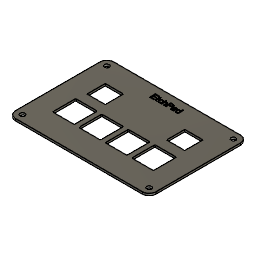
EtchPad_Case (Autodesk Fusion 360 archive; units mm, degrees)
design "EtchPad_Case_Top"
Autodesk Fusion 360 part; units mm, degrees
sketch "Sketch1" plane through (0, 0, 0) normal (0, 0, 1) x (1, 0, 0)
  line L0 (3.025, -31.1) -> (16.025, -31.1)
  line L1 (3.025, -45.1) -> (16.025, -45.1)
  line L2 (2.525, -31.6) -> (2.525, -44.6)
  line L3 (16.525, -31.6) -> (16.525, -44.6)
  arc A0 (3.025, -31.1) -> (2.525, -31.6) centre (3.025, -31.6) ccw
  arc A1 (16.525, -31.6) -> (16.025, -31.1) centre (16.025, -31.6) ccw
  arc A2 (2.525, -44.6) -> (3.025, -45.1) centre (3.025, -44.6) ccw
  arc A3 (16.025, -45.1) -> (16.525, -44.6) centre (16.025, -44.6) ccw
  line L4 (22.075, -31.1) -> (35.075, -31.1)
  line L5 (22.075, -45.1) -> (35.075, -45.1)
  line L6 (21.575, -31.6) -> (21.575, -44.6)
  line L7 (35.575, -31.6) -> (35.575, -44.6)
  arc A4 (22.075, -31.1) -> (21.575, -31.6) centre (22.075, -31.6) ccw
  arc A5 (35.575, -31.6) -> (35.075, -31.1) centre (35.075, -31.6) ccw
  arc A6 (21.575, -44.6) -> (22.075, -45.1) centre (22.075, -44.6) ccw
  arc A7 (35.075, -45.1) -> (35.575, -44.6) centre (35.075, -44.6) ccw
  line L8 (41.125, -31.1) -> (54.125, -31.1)
  line L9 (41.125, -45.1) -> (54.125, -45.1)
  line L10 (40.625, -31.6) -> (40.625, -44.6)
  line L11 (54.625, -31.6) -> (54.625, -44.6)
  arc A8 (41.125, -31.1) -> (40.625, -31.6) centre (41.125, -31.6) ccw
  arc A9 (54.625, -31.6) -> (54.125, -31.1) centre (54.125, -31.6) ccw
  arc A10 (40.625, -44.6) -> (41.125, -45.1) centre (41.125, -44.6) ccw
  arc A11 (54.125, -45.1) -> (54.625, -44.6) centre (54.125, -44.6) ccw
  line L12 (60.175, -31.1) -> (73.175, -31.1)
  line L13 (60.175, -45.1) -> (73.175, -45.1)
  line L14 (59.675, -31.6) -> (59.675, -44.6)
  line L15 (73.675, -31.6) -> (73.675, -44.6)
  arc A12 (60.175, -31.1) -> (59.675, -31.6) centre (60.175, -31.6) ccw
  arc A13 (73.675, -31.6) -> (73.175, -31.1) centre (73.175, -31.6) ccw
  arc A14 (59.675, -44.6) -> (60.175, -45.1) centre (60.175, -44.6) ccw
  arc A15 (73.175, -45.1) -> (73.675, -44.6) centre (73.175, -44.6) ccw
  line L16 (88.6, -63.6) -> (-12.4, -63.6)
  line L17 (-12.4, -63.6) -> (-12.4, 7)
  line L18 (-12.4, 7) -> (88.6, 7)
  line L19 (88.6, 7) -> (88.6, -63.6)
  line L20 (88.6, -63.6) -> (-12.4, 7) construction
  line L21 (-12.4, -63.6) -> (88.6, 7) construction
  line L22 (78.6, -53.6) -> (-2.4, -53.6)
  line L23 (-2.4, -53.6) -> (-2.4, -3)
  line L24 (-2.4, -3) -> (78.6, -3)
  line L25 (78.6, -3) -> (78.6, -53.6)
  circle A16 centre (-7.4, -58.6) radius 1.7
  circle A17 centre (83.6, 2) radius 1.7
  circle A18 centre (83.6, -58.6) radius 1.7
  circle A19 centre (-7.4, 2) radius 1.7
  point P0 (38.1, -28.3)
  dimension "d1" = 101
  dimension "d2" = 70.6
  dimension "d3" = 10
  dimension "d9" = 3.4
  dimension "d12" = 3.4
  dimension "d13" = 3.4
  dimension "d14" = 3.4
  constraint horizontal L16
  constraint perpendicular L16 L17
  constraint parallel L16 L18
  constraint parallel L17 L19
  constraint coincident L20 P0
  constraint coincident L21 P0
  measures "d1" distance of L17.end L18.end
  measures "d2" distance of L16.end L17.end
  measures "d9" diameter of A16
  measures "d12" diameter of A17
  measures "d13" diameter of A18
  measures "d14" diameter of A19
extrude "Extrude1" add sketch "Sketch1" along normal blind 1.5 contours L16 L17 L18 L19 | L22 L23 L24 L25
sketch "Sketch2" plane through (0, 0, 1.5) normal (0, 0, 1) x (-1, 0, 0)
  arc A0 (-41.125, 31.1) -> (-40.625, 31.6) centre (-41.125, 31.6) ccw
  line L0 (-41.125, 31.1) -> (-54.125, 31.1)
  arc A1 (-54.625, 31.6) -> (-54.125, 31.1) centre (-54.125, 31.6) ccw
  line L1 (-54.625, 31.6) -> (-54.625, 44.6)
  arc A2 (-54.125, 45.1) -> (-54.625, 44.6) centre (-54.125, 44.6) ccw
  line L2 (-54.125, 45.1) -> (-41.125, 45.1)
  arc A3 (-40.625, 44.6) -> (-41.125, 45.1) centre (-41.125, 44.6) ccw
  line L3 (-40.625, 44.6) -> (-40.625, 31.6)
  circle A4 centre (-83.6, 58.6) radius 1.7
  circle A5 centre (7.4, 58.6) radius 1.7
  arc A6 (-22.075, 31.1) -> (-21.575, 31.6) centre (-22.075, 31.6) ccw
  line L4 (-22.075, 31.1) -> (-35.075, 31.1)
  arc A7 (-35.575, 31.6) -> (-35.075, 31.1) centre (-35.075, 31.6) ccw
  line L5 (-35.575, 31.6) -> (-35.575, 44.6)
  arc A8 (-35.075, 45.1) -> (-35.575, 44.6) centre (-35.075, 44.6) ccw
  line L6 (-35.075, 45.1) -> (-22.075, 45.1)
  arc A9 (-21.575, 44.6) -> (-22.075, 45.1) centre (-22.075, 44.6) ccw
  line L7 (-21.575, 44.6) -> (-21.575, 31.6)
  arc A10 (-3.025, 31.1) -> (-2.525, 31.6) centre (-3.025, 31.6) ccw
  line L8 (-3.025, 31.1) -> (-16.025, 31.1)
  arc A11 (-16.525, 31.6) -> (-16.025, 31.1) centre (-16.025, 31.6) ccw
  line L9 (-16.525, 31.6) -> (-16.525, 44.6)
  arc A12 (-16.025, 45.1) -> (-16.525, 44.6) centre (-16.025, 44.6) ccw
  line L10 (-16.025, 45.1) -> (-3.025, 45.1)
  arc A13 (-2.525, 44.6) -> (-3.025, 45.1) centre (-3.025, 44.6) ccw
  line L11 (-2.525, 44.6) -> (-2.525, 31.6)
  arc A14 (-60.175, 31.1) -> (-59.675, 31.6) centre (-60.175, 31.6) ccw
  line L12 (-60.175, 31.1) -> (-73.175, 31.1)
  arc A15 (-73.675, 31.6) -> (-73.175, 31.1) centre (-73.175, 31.6) ccw
  line L13 (-73.675, 31.6) -> (-73.675, 44.6)
  arc A16 (-73.175, 45.1) -> (-73.675, 44.6) centre (-73.175, 44.6) ccw
  line L14 (-73.175, 45.1) -> (-60.175, 45.1)
  arc A17 (-59.675, 44.6) -> (-60.175, 45.1) centre (-60.175, 44.6) ccw
  line L15 (-59.675, 44.6) -> (-59.675, 31.6)
  circle A18 centre (-83.6, -2) radius 1.7
  circle A19 centre (7.4, -2) radius 1.7
  line L16 (-88.6, -7) -> (12.4, -7)
  line L17 (12.4, -7) -> (12.4, 63.6)
  line L18 (12.4, 63.6) -> (-88.6, 63.6)
  line L19 (-88.6, 63.6) -> (-88.6, -7)
  line L20 (-27.4431, 12.4012) -> (-48.7413, 12.4127) construction
  line L21 (-48.7413, 12.4127) -> (-48.7491, -1.9941) construction
  line L22 (-48.7491, -1.9941) -> (-27.4509, -2.0057) construction
  line L23 (-27.4509, -2.0057) -> (-27.4431, 12.4012) construction
  line L24 (-38.1, -2) -> (-38.1, -1.9999)
  dimension "d17" = 4
  dimension "d20" = 0.0001
  text T0 "EtchPad" font "Arial" height 4 align left top in box 21.2982 x 14.4068 at (-27.4431, 12.4012) x (-1, 0.000542) y (-0.000542, -1) spacing 1 kerned
  constraint midpoint L22 L24.end
  constraint vertical L24
  measures "d20" distance of L24.start L24.end
extrude "Extrude2" cut sketch "Sketch2" against normal blind 0.2 text T0
fillet "Fillet1" radius 5 4 edges at (-12.4, -63.6, 0.75) (88.6, -63.6, 0.75) (88.6, 7, 0.75) (-12.4, 7, 0.75)
sketch "Sketch3" plane through (0, 0, 1.5) normal (0, 0, 1) x (-1, 0, 0)
  arc A0 (7.4, -7) -> (12.4, -2) centre (7.4, -2) ccw
  line L0 (12.4, -2) -> (12.4, 58.6)
  arc A1 (12.4, 58.6) -> (7.4, 63.6) centre (7.4, 58.6) ccw
  line L1 (7.4, 63.6) -> (-83.6, 63.6)
  arc A2 (-83.6, 63.6) -> (-88.6, 58.6) centre (-83.6, 58.6) ccw
  line L2 (-88.6, 58.6) -> (-88.6, -2)
  arc A3 (-88.6, -2) -> (-83.6, -7) centre (-83.6, -2) ccw
  line L3 (-83.6, -7) -> (7.4, -7)
  circle A4 centre (7.4, -2) radius 1.7
  circle A5 centre (-83.6, -2) radius 1.7
  arc A6 (-60.175, 31.1) -> (-59.675, 31.6) centre (-60.175, 31.6) ccw
  line L4 (-60.175, 31.1) -> (-73.175, 31.1)
  arc A7 (-73.675, 31.6) -> (-73.175, 31.1) centre (-73.175, 31.6) ccw
  line L5 (-73.675, 31.6) -> (-73.675, 44.6)
  arc A8 (-73.175, 45.1) -> (-73.675, 44.6) centre (-73.175, 44.6) ccw
  line L6 (-73.175, 45.1) -> (-60.175, 45.1)
  arc A9 (-59.675, 44.6) -> (-60.175, 45.1) centre (-60.175, 44.6) ccw
  line L7 (-59.675, 44.6) -> (-59.675, 31.6)
  arc A10 (-3.025, 31.1) -> (-2.525, 31.6) centre (-3.025, 31.6) ccw
  line L8 (-3.025, 31.1) -> (-16.025, 31.1)
  arc A11 (-16.525, 31.6) -> (-16.025, 31.1) centre (-16.025, 31.6) ccw
  line L9 (-16.525, 31.6) -> (-16.525, 44.6)
  arc A12 (-16.025, 45.1) -> (-16.525, 44.6) centre (-16.025, 44.6) ccw
  line L10 (-16.025, 45.1) -> (-3.025, 45.1)
  arc A13 (-2.525, 44.6) -> (-3.025, 45.1) centre (-3.025, 44.6) ccw
  line L11 (-2.525, 44.6) -> (-2.525, 31.6)
  arc A14 (-22.075, 31.1) -> (-21.575, 31.6) centre (-22.075, 31.6) ccw
  line L12 (-22.075, 31.1) -> (-35.075, 31.1)
  arc A15 (-35.575, 31.6) -> (-35.075, 31.1) centre (-35.075, 31.6) ccw
  line L13 (-35.575, 31.6) -> (-35.575, 44.6)
  arc A16 (-35.075, 45.1) -> (-35.575, 44.6) centre (-35.075, 44.6) ccw
  line L14 (-35.075, 45.1) -> (-22.075, 45.1)
  arc A17 (-21.575, 44.6) -> (-22.075, 45.1) centre (-22.075, 44.6) ccw
  line L15 (-21.575, 44.6) -> (-21.575, 31.6)
  circle A18 centre (7.4, 58.6) radius 1.7
  circle A19 centre (-83.6, 58.6) radius 1.7
  arc A20 (-41.125, 31.1) -> (-40.625, 31.6) centre (-41.125, 31.6) ccw
  line L16 (-41.125, 31.1) -> (-54.125, 31.1)
  arc A21 (-54.625, 31.6) -> (-54.125, 31.1) centre (-54.125, 31.6) ccw
  line L17 (-54.625, 31.6) -> (-54.625, 44.6)
  arc A22 (-54.125, 45.1) -> (-54.625, 44.6) centre (-54.125, 44.6) ccw
  line L18 (-54.125, 45.1) -> (-41.125, 45.1)
  arc A23 (-40.625, 44.6) -> (-41.125, 45.1) centre (-41.125, 44.6) ccw
  line L19 (-40.625, 44.6) -> (-40.625, 31.6)
  line L20 (-30.434, 1.5239) -> (-30.4337, 1.9959)
  line L21 (-30.4337, 1.9959) -> (-27.4487, 1.9943)
  line L22 (-27.4487, 1.9943) -> (-27.4509, -2.0057)
  line L23 (-27.4509, -2.0057) -> (-30.3431, -2.0041)
  line L24 (-30.3431, -2.0041) -> (-30.3429, -1.5321)
  line L25 (-30.3429, -1.5321) -> (-27.98, -1.5334)
  line L26 (-27.98, -1.5334) -> (-27.9793, -0.3083)
  line L27 (-27.9793, -0.3083) -> (-30.1921, -0.3071)
  line L28 (-30.1921, -0.3071) -> (-30.1919, 0.1623)
  line L29 (-30.1919, 0.1623) -> (-27.979, 0.1611)
  line L30 (-27.979, 0.1611) -> (-27.9783, 1.5226)
  line L31 (-27.9783, 1.5226) -> (-30.434, 1.5239)
  spline S0 degree 3 poles (-33.8172, 1.6594) (-33.9088, 1.6529) (-34.087, 1.6402) (-34.2305, 1.534) (-34.3003, 1.4824) knots 0 0 0 0 0.026903 0.052406 0.052406 0.052406 0.052406
  spline S1 degree 3 poles (-34.3003, 1.4824) (-34.3596, 1.4104) (-34.4904, 1.2516) (-34.5265, 1.0481) (-34.5462, 0.9368) knots 0 0 0 0 0.027516 0.060744 0.060744 0.060744 0.060744
  line L32 (-34.5462, 0.9368) -> (-35.0291, 0.9998)
  spline S2 degree 3 poles (-35.0291, 0.9998) (-34.9949, 1.1549) (-34.9293, 1.4522) (-34.7224, 1.6748) (-34.6235, 1.7813) knots 0 0 0 0 0.046685 0.089485 0.089485 0.089485 0.089485
  spline S3 degree 3 poles (-34.6235, 1.7813) (-34.5065, 1.8636) (-34.2664, 2.0326) (-33.973, 2.0529) (-33.8225, 2.0633) knots 0 0 0 0 0.042047 0.086372 0.086372 0.086372 0.086372
  spline S4 degree 3 poles (-33.8225, 2.0633) (-33.636, 2.0492) (-33.2748, 2.0218) (-32.9995, 1.7874) (-32.8664, 1.6739) knots 0 0 0 0 0.054523 0.105641 0.105641 0.105641 0.105641
  spline S5 degree 3 poles (-32.8664, 1.6739) (-32.7612, 1.5213) (-32.5311, 1.1873) (-32.5145, 0.7802) (-32.5054, 0.5591) knots 0 0 0 0 0.054525 0.119313 0.119313 0.119313 0.119313
  spline S6 degree 3 poles (-32.5054, 0.5591) (-32.5106, 0.4109) (-32.5203, 0.129) (-32.616, -0.1362) (-32.6614, -0.2621) knots 0 0 0 0 0.044169 0.084044 0.084044 0.084044 0.084044
  spline S7 degree 3 poles (-32.6614, -0.2621) (-32.7192, -0.3715) (-32.8331, -0.5872) (-33.0355, -0.7229) (-33.1351, -0.7898) knots 0 0 0 0 0.036512 0.071907 0.071907 0.071907 0.071907
  spline S8 degree 3 poles (-33.1351, -0.7898) (-33.2439, -0.841) (-33.463, -0.9443) (-33.705, -0.9583) (-33.8269, -0.9654) knots 0 0 0 0 0.035714 0.071964 0.071964 0.071964 0.071964
  spline S9 degree 3 poles (-33.8269, -0.9654) (-33.9738, -0.9578) (-34.2521, -0.9434) (-34.4877, -0.7959) (-34.5989, -0.7262) knots 0 0 0 0 0.043319 0.082021 0.082021 0.082021 0.082021
  spline S10 degree 3 poles (-34.5989, -0.7262) (-34.6904, -0.6354) (-34.8816, -0.4456) (-34.9484, -0.1842) (-34.9833, -0.048) knots 0 0 0 0 0.037959 0.079265 0.079265 0.079265 0.079265
  line L33 (-34.9833, -0.048) -> (-34.5057, 0.0254)
  spline S11 degree 3 poles (-34.5057, 0.0254) (-34.4811, -0.0637) (-34.4352, -0.2297) (-34.3185, -0.3557) (-34.2645, -0.414) knots 0 0 0 0 0.027269 0.05078 0.05078 0.05078 0.05078
  spline S12 degree 3 poles (-34.2645, -0.414) (-34.2029, -0.457) (-34.0771, -0.5448) (-33.9239, -0.5559) (-33.8457, -0.5616) knots 0 0 0 0 0.022095 0.045141 0.045141 0.045141 0.045141
  spline S13 degree 3 poles (-33.8457, -0.5616) (-33.7284, -0.5512) (-33.4971, -0.5307) (-33.3266, -0.3734) (-33.2426, -0.2958) knots 0 0 0 0 0.03428 0.067589 0.067589 0.067589 0.067589
  spline S14 degree 3 poles (-33.2426, -0.2958) (-33.1752, -0.1842) (-33.0199, 0.0729) (-33.0137, 0.3749) (-33.0102, 0.5458) knots 0 0 0 0 0.038499 0.088664 0.088664 0.088664 0.088664
  spline S15 degree 3 poles (-33.0102, 0.5458) (-33.013, 0.7184) (-33.0179, 1.0214) (-33.1686, 1.2822) (-33.2335, 1.3945) knots 0 0 0 0 0.050719 0.089036 0.089036 0.089036 0.089036
  spline S16 degree 3 poles (-33.2335, 1.3945) (-33.3144, 1.4717) (-33.4779, 1.6279) (-33.7033, 1.6489) (-33.8172, 1.6594) knots 0 0 0 0 0.03254 0.06581 0.06581 0.06581 0.06581
  line L34 (-35.9407, 0.4137) -> (-35.9398, 1.9989)
  line L35 (-35.9398, 1.9989) -> (-35.4487, 1.9987)
  line L36 (-35.4487, 1.9987) -> (-35.4509, -2.0013)
  line L37 (-35.4509, -2.0013) -> (-35.942, -2.0011)
  line L38 (-35.942, -2.0011) -> (-35.9412, -0.5659)
  spline S17 degree 3 poles (-35.9412, -0.5659) (-36.0633, -0.682) (-36.3071, -0.9139) (-36.6419, -0.9472) (-36.8091, -0.9638) knots 0 0 0 0 0.049035 0.097945 0.097945 0.097945 0.097945
  spline S18 degree 3 poles (-36.8091, -0.9638) (-36.9109, -0.9595) (-37.1053, -0.9513) (-37.2835, -0.8736) (-37.3684, -0.8366) knots 0 0 0 0 0.030249 0.057797 0.057797 0.057797 0.057797
  spline S19 degree 3 poles (-37.3684, -0.8366) (-37.4414, -0.7912) (-37.584, -0.7025) (-37.6673, -0.5568) (-37.7079, -0.4858) knots 0 0 0 0 0.025355 0.049506 0.049506 0.049506 0.049506
  spline S20 degree 3 poles (-37.7079, -0.4858) (-37.7376, -0.3951) (-37.8064, -0.1846) (-37.8086, 0.0374) (-37.8099, 0.1637) knots 0 0 0 0 0.028475 0.066079 0.066079 0.066079 0.066079
  line L39 (-37.8099, 0.1637) -> (-37.8089, 1.9999)
  line L40 (-37.8089, 1.9999) -> (-37.3177, 1.9997)
  line L41 (-37.3177, 1.9997) -> (-37.3187, 0.1634)
  spline S21 degree 3 poles (-37.3187, 0.1634) (-37.3163, 0.0538) (-37.3118, -0.1407) (-37.2057, -0.3023) (-37.1594, -0.3729) knots 0 0 0 0 0.032071 0.056936 0.056936 0.056936 0.056936
  spline S22 degree 3 poles (-37.1594, -0.3729) (-37.0979, -0.4218) (-36.9663, -0.5264) (-36.7977, -0.5359) (-36.7079, -0.5409) knots 0 0 0 0 0.023016 0.04924 0.04924 0.04924 0.04924
  spline S23 degree 3 poles (-36.7079, -0.5409) (-36.6361, -0.5361) (-36.4915, -0.5265) (-36.3622, -0.4609) (-36.2972, -0.4279) knots 0 0 0 0 0.021368 0.04299 0.04299 0.04299 0.04299
  spline S24 degree 3 poles (-36.2972, -0.4279) (-36.2379, -0.3874) (-36.1212, -0.3076) (-36.0553, -0.1826) (-36.0229, -0.1211) knots 0 0 0 0 0.021195 0.041719 0.041719 0.041719 0.041719
  spline S25 degree 3 poles (-36.0229, -0.1211) (-35.999, -0.0448) (-35.9448, 0.129) (-35.9422, 0.3114) (-35.9407, 0.4137) knots 0 0 0 0 0.023859 0.054351 0.054351 0.054351 0.054351
  line L42 (-44.7857, 2.0037) -> (-44.2727, 2.0034)
  spline S26 degree 3 poles (-44.2727, 2.0034) (-44.2494, 1.9489) (-44.2005, 1.8342) (-44.1836, 1.7107) (-44.1747, 1.646) knots 0 0 0 0 0.017724 0.037217 0.037217 0.037217 0.037217
  spline S27 degree 3 poles (-44.1747, 1.646) (-44.0881, 1.7162) (-43.9264, 1.8471) (-43.7371, 1.9332) (-43.6493, 1.9731) knots 0 0 0 0 0.033289 0.062117 0.062117 0.062117 0.062117
  spline S28 degree 3 poles (-43.6493, 1.9731) (-43.5628, 2.0009) (-43.3866, 2.0575) (-43.2017, 2.0647) (-43.1076, 2.0683) knots 0 0 0 0 0.027122 0.055225 0.055225 0.055225 0.055225
  spline S29 degree 3 poles (-43.1076, 2.0683) (-42.9623, 2.0624) (-42.6951, 2.0516) (-42.4744, 1.9026) (-42.3738, 1.8346) knots 0 0 0 0 0.042625 0.078372 0.078372 0.078372 0.078372
  spline S30 degree 3 poles (-42.3738, 1.8346) (-42.299, 1.7506) (-42.1475, 1.5805) (-42.1277, 1.3533) (-42.1176, 1.2383) knots 0 0 0 0 0.032801 0.066467 0.066467 0.066467 0.066467
  spline S31 degree 3 poles (-42.1176, 1.2383) (-42.1214, 1.1693) (-42.129, 1.0335) (-42.1864, 0.9102) (-42.2147, 0.8495) knots 0 0 0 0 0.020505 0.040399 0.040399 0.040399 0.040399
  spline S32 degree 3 poles (-42.2147, 0.8495) (-42.2491, 0.7941) (-42.3169, 0.6848) (-42.4185, 0.606) (-42.4686, 0.5673) knots 0 0 0 0 0.019408 0.038238 0.038238 0.038238 0.038238
  spline S33 degree 3 poles (-42.4686, 0.5673) (-42.5231, 0.5338) (-42.6343, 0.4657) (-42.7587, 0.4265) (-42.822, 0.4065) knots 0 0 0 0 0.019118 0.038959 0.038959 0.038959 0.038959
  spline S34 degree 3 poles (-42.822, 0.4065) (-42.8824, 0.3932) (-43.0266, 0.3615) (-43.1733, 0.3435) (-43.2586, 0.333) knots 0 0 0 0 0.018529 0.044295 0.044295 0.044295 0.044295
  spline S35 degree 3 poles (-43.2586, 0.333) (-43.4318, 0.3122) (-43.7279, 0.2765) (-44.0152, 0.1973) (-44.1346, 0.1644) knots 0 0 0 0 0.052219 0.089311 0.089311 0.089311 0.089311
  spline S36 degree 3 poles (-44.1346, 0.1644) (-44.1354, 0.1368) (-44.1366, 0.0941) (-44.1372, 0.0514) (-44.1374, 0.0361) knots 0 0 0 0 0.008256 0.012827 0.012827 0.012827 0.012827
  spline S37 degree 3 poles (-44.1374, 0.0361) (-44.1355, -0.0526) (-44.1321, -0.2091) (-44.0388, -0.3332) (-43.9984, -0.3869) knots 0 0 0 0 0.025815 0.045519 0.045519 0.045519 0.045519
  spline S38 degree 3 poles (-43.9984, -0.3869) (-43.9226, -0.4353) (-43.7531, -0.5437) (-43.551, -0.5501) (-43.4392, -0.5536) knots 0 0 0 0 0.026519 0.059321 0.059321 0.059321 0.059321
  spline S39 degree 3 poles (-43.4392, -0.5536) (-43.3366, -0.5521) (-43.1563, -0.5494) (-42.9964, -0.4677) (-42.9275, -0.4325) knots 0 0 0 0 0.030269 0.053198 0.053198 0.053198 0.053198
  spline S40 degree 3 poles (-42.9275, -0.4325) (-42.8749, -0.3793) (-42.7556, -0.2586) (-42.7091, -0.0946) (-42.6831, -0.0029) knots 0 0 0 0 0.022111 0.050139 0.050139 0.050139 0.050139
  line L43 (-42.6831, -0.0029) -> (-42.2029, -0.0686)
  spline S41 degree 3 poles (-42.2029, -0.0686) (-42.2264, -0.1639) (-42.2703, -0.3422) (-42.3716, -0.4952) (-42.4187, -0.5665) knots 0 0 0 0 0.029181 0.05462 0.05462 0.05462 0.05462
  spline S42 degree 3 poles (-42.4187, -0.5665) (-42.4768, -0.6269) (-42.6003, -0.7551) (-42.7654, -0.8225) (-42.8527, -0.8582) knots 0 0 0 0 0.024865 0.052809 0.052809 0.052809 0.052809
  spline S43 degree 3 poles (-42.8527, -0.8582) (-42.9542, -0.8879) (-43.1687, -0.9509) (-43.3924, -0.9569) (-43.5103, -0.9601) knots 0 0 0 0 0.031574 0.066797 0.066797 0.066797 0.066797
  spline S44 degree 3 poles (-43.5103, -0.9601) (-43.6233, -0.9582) (-43.8282, -0.9546) (-44.025, -0.8979) (-44.1133, -0.8725) knots 0 0 0 0 0.0337 0.061163 0.061163 0.061163 0.061163
  spline S45 degree 3 poles (-44.1133, -0.8725) (-44.1833, -0.844) (-44.311, -0.792) (-44.4096, -0.696) (-44.4542, -0.6527) knots 0 0 0 0 0.022407 0.040904 0.040904 0.040904 0.040904
  spline S46 degree 3 poles (-44.4542, -0.6527) (-44.4882, -0.6041) (-44.5595, -0.5022) (-44.5906, -0.3816) (-44.6069, -0.3183) knots 0 0 0 0 0.017614 0.037017 0.037017 0.037017 0.037017
  spline S47 degree 3 poles (-44.6069, -0.3183) (-44.6139, -0.2597) (-44.632, -0.1094) (-44.6315, 0.0422) (-44.6312, 0.1346) knots 0 0 0 0 0.017695 0.045396 0.045396 0.045396 0.045396
  line L44 (-44.6312, 0.1346) -> (-44.6308, 0.7895)
  spline S48 degree 3 poles (-44.6308, 0.7895) (-44.6296, 0.976) (-44.6277, 1.2653) (-44.6528, 1.5534) (-44.6617, 1.6558) knots 0 0 0 0 0.055906 0.086726 0.086726 0.086726 0.086726
  spline S49 degree 3 poles (-44.6617, 1.6558) (-44.6748, 1.7159) (-44.7013, 1.8371) (-44.7574, 1.9479) (-44.7857, 2.0037) knots 0 0 0 0 0.018374 0.037071 0.037071 0.037071 0.037071
  line L45 (-39.1495, 0.3745) -> (-39.1486, 2.0007)
  line L46 (-39.1486, 2.0007) -> (-38.6192, 2.0004)
  line L47 (-38.6192, 2.0004) -> (-38.6214, -1.9996)
  line L48 (-38.6214, -1.9996) -> (-40.1303, -1.9988)
  spline S50 degree 3 poles (-40.1303, -1.9988) (-40.2476, -1.9984) (-40.4512, -1.9976) (-40.6531, -1.9714) (-40.7387, -1.9603) knots 0 0 0 0 0.035143 0.061018 0.061018 0.061018 0.061018
  spline S51 degree 3 poles (-40.7387, -1.9603) (-40.8309, -1.9415) (-41.0059, -1.9059) (-41.1597, -1.8158) (-41.2325, -1.7731) knots 0 0 0 0 0.028003 0.053127 0.053127 0.053127 0.053127
  spline S52 degree 3 poles (-41.2325, -1.7731) (-41.2963, -1.7212) (-41.4284, -1.6136) (-41.5104, -1.4642) (-41.5529, -1.3868) knots 0 0 0 0 0.024427 0.050607 0.050607 0.050607 0.050607
  spline S53 degree 3 poles (-41.5529, -1.3868) (-41.5882, -1.3011) (-41.6603, -1.1263) (-41.6694, -0.9373) (-41.674, -0.8411) knots 0 0 0 0 0.027603 0.056277 0.056277 0.056277 0.056277
  spline S54 degree 3 poles (-41.674, -0.8411) (-41.6613, -0.6786) (-41.6364, -0.359) (-41.4436, -0.1033) (-41.3488, 0.0223) knots 0 0 0 0 0.047795 0.093992 0.093992 0.093992 0.093992
  spline S55 degree 3 poles (-41.3488, 0.0223) (-41.2016, 0.1247) (-40.8525, 0.3674) (-40.4235, 0.3722) (-40.1754, 0.375) knots 0 0 0 0 0.052712 0.125014 0.125014 0.125014 0.125014
  line L49 (-40.1754, 0.375) -> (-39.1495, 0.3745)
  line L50 (-47.7292, -1.9947) -> (-47.727, 2.0053)
  line L51 (-47.727, 2.0053) -> (-47.2714, 2.0051)
  line L52 (-47.2714, 2.0051) -> (-47.2716, 1.6395)
  spline S56 degree 3 poles (-47.2716, 1.6395) (-47.1677, 1.7651) (-46.9571, 2.0199) (-46.6278, 2.0532) (-46.461, 2.0701) knots 0 0 0 0 0.046947 0.095166 0.095166 0.095166 0.095166
  spline S57 degree 3 poles (-46.461, 2.0701) (-46.3477, 2.0621) (-46.1211, 2.046) (-45.9231, 1.9345) (-45.824, 1.8788) knots 0 0 0 0 0.033595 0.067252 0.067252 0.067252 0.067252
  spline S58 degree 3 poles (-45.824, 1.8788) (-45.732, 1.8075) (-45.5441, 1.6619) (-45.4315, 1.4522) (-45.374, 1.3451) knots 0 0 0 0 0.034476 0.070499 0.070499 0.070499 0.070499
  spline S59 degree 3 poles (-45.374, 1.3451) (-45.3276, 1.2238) (-45.2305, 0.9705) (-45.2202, 0.6992) (-45.2148, 0.5578) knots 0 0 0 0 0.038699 0.080805 0.080805 0.080805 0.080805
  spline S60 degree 3 poles (-45.2148, 0.5578) (-45.2201, 0.4187) (-45.2303, 0.1491) (-45.3177, -0.1059) (-45.3599, -0.2293) knots 0 0 0 0 0.041529 0.080418 0.080418 0.080418 0.080418
  spline S61 degree 3 poles (-45.3599, -0.2293) (-45.4128, -0.3392) (-45.5159, -0.5534) (-45.703, -0.6995) (-45.794, -0.7706) knots 0 0 0 0 0.036065 0.070231 0.070231 0.070231 0.070231
  spline S62 degree 3 poles (-45.794, -0.7706) (-45.8938, -0.8255) (-46.0954, -0.9362) (-46.3249, -0.9511) (-46.4408, -0.9585) knots 0 0 0 0 0.033726 0.068088 0.068088 0.068088 0.068088
  spline S63 degree 3 poles (-46.4408, -0.9585) (-46.5246, -0.9545) (-46.6871, -0.9466) (-46.8354, -0.88) (-46.9073, -0.8478) knots 0 0 0 0 0.024915 0.048327 0.048327 0.048327 0.048327
  spline S64 degree 3 poles (-46.9073, -0.8478) (-46.9719, -0.8086) (-47.0993, -0.7315) (-47.1936, -0.6164) (-47.24, -0.5597) knots 0 0 0 0 0.022496 0.044294 0.044294 0.044294 0.044294
  line L53 (-47.24, -0.5597) -> (-47.2408, -1.9949)
  line L54 (-47.2408, -1.9949) -> (-47.7292, -1.9947)
  spline S65 degree 3 poles (-31.7914, 1.541) (-31.8148, 1.5513) (-31.8681, 1.5748) (-31.9265, 1.5759) (-31.9592, 1.5766) knots 0 0 0 0 0.007608 0.017301 0.017301 0.017301 0.017301
  spline S66 degree 3 poles (-31.9592, 1.5766) (-31.9908, 1.5755) (-32.063, 1.573) (-32.1346, 1.5631) (-32.1747, 1.5576) knots 0 0 0 0 0.009494 0.021652 0.021652 0.021652 0.021652
  line L55 (-32.1747, 1.5576) -> (-32.2454, 1.9915)
  spline S67 degree 3 poles (-32.2454, 1.9915) (-32.1802, 2.0042) (-32.0575, 2.028) (-31.9327, 2.0327) (-31.8743, 2.0349) knots 0 0 0 0 0.019916 0.037413 0.037413 0.037413 0.037413
  spline S68 degree 3 poles (-31.8743, 2.0349) (-31.794, 2.0333) (-31.6502, 2.0305) (-31.518, 1.9747) (-31.4597, 1.9501) knots 0 0 0 0 0.023832 0.042668 0.042668 0.042668 0.042668
  spline S69 degree 3 poles (-31.4597, 1.9501) (-31.4146, 1.9205) (-31.3272, 1.8631) (-31.2768, 1.7718) (-31.2524, 1.7276) knots 0 0 0 0 0.015917 0.030816 0.030816 0.030816 0.030816
  spline S70 degree 3 poles (-31.2524, 1.7276) (-31.2352, 1.6566) (-31.1891, 1.4666) (-31.1913, 1.2706) (-31.1927, 1.1478) knots 0 0 0 0 0.021853 0.05848 0.05848 0.05848 0.05848
  line L56 (-31.1927, 1.1478) -> (-31.1936, -0.5193)
  line L57 (-31.1936, -0.5193) -> (-30.8334, -0.5195)
  line L58 (-30.8334, -0.5195) -> (-30.8336, -0.9015)
  line L59 (-30.8336, -0.9015) -> (-31.1938, -0.9013)
  line L60 (-31.1938, -0.9013) -> (-31.1942, -1.6189)
  line L61 (-31.1942, -1.6189) -> (-31.6828, -1.9133)
  line L62 (-31.6828, -1.9133) -> (-31.6822, -0.9011)
  line L63 (-31.6822, -0.9011) -> (-32.1761, -0.9008)
  line L64 (-32.1761, -0.9008) -> (-32.1759, -0.5188)
  line L65 (-32.1759, -0.5188) -> (-31.682, -0.5191)
  line L66 (-31.682, -0.5191) -> (-31.6811, 1.1753)
  spline S71 degree 3 poles (-31.6811, 1.1753) (-31.6803, 1.2332) (-31.6791, 1.3244) (-31.6994, 1.4131) (-31.7069, 1.4455) knots 0 0 0 0 0.01727 0.027216 0.027216 0.027216 0.027216
  spline S72 degree 3 poles (-31.7069, 1.4455) (-31.717, 1.4645) (-31.7375, 1.5032) (-31.7733, 1.5283) (-31.7914, 1.541) knots 0 0 0 0 0.006377 0.012919 0.012919 0.012919 0.012919
  line L67 (-28.575, 38.1) -> (-28.575, 50.1)
  line L68 (-47.625, 38.1) -> (-47.625, 50.1)
  line L69 (-66.675, 38.1) -> (-66.675, 50.1)
  circle A24 centre (-9.525, 50.1) radius 1.75
  circle A25 centre (-28.575, 50.1) radius 1.75
  circle A26 centre (-47.625, 50.1) radius 1.75
  circle A27 centre (-66.675, 50.1) radius 1.75
  line L70 (-9.525, 31.1) -> (-9.525, 29.6)
  line L71 (-9.525, 45.1) -> (-9.525, 46.1)
  line L72 (-16.525, 38.1) -> (-17.275, 38.1)
  line L73 (-2.525, 38.1) -> (-1.775, 38.1)
  line L74 (-2.275, 29.6) -> (-16.775, 29.6)
  line L75 (-17.275, 30.1) -> (-17.275, 45.6)
  line L76 (-16.775, 46.1) -> (-2.275, 46.1)
  line L77 (-1.775, 45.6) -> (-1.775, 30.1)
  line L78 (-35.825, 46.35) -> (-21.325, 46.35)
  line L79 (-20.825, 45.85) -> (-20.825, 30.35)
  line L80 (-21.325, 29.85) -> (-35.825, 29.85)
  line L81 (-36.325, 30.35) -> (-36.325, 45.85)
  line L82 (-54.875, 46.35) -> (-40.375, 46.35)
  line L83 (-39.875, 45.85) -> (-39.875, 30.35)
  line L84 (-40.375, 29.85) -> (-54.875, 29.85)
  line L85 (-55.375, 30.35) -> (-55.375, 45.85)
  line L86 (-73.925, 46.35) -> (-59.425, 46.35)
  line L87 (-58.925, 45.85) -> (-58.925, 30.35)
  line L88 (-59.425, 29.85) -> (-73.925, 29.85)
  line L89 (-74.425, 30.35) -> (-74.425, 45.85)
  circle A28 centre (-9.525, 19.4) radius 6
  circle A29 centre (-66.675, 19.4) radius 6
  arc A30 (-21.325, 29.85) -> (-20.825, 30.35) centre (-21.325, 30.35) ccw
  arc A31 (-36.325, 30.35) -> (-35.825, 29.85) centre (-35.825, 30.35) ccw
  arc A32 (-35.825, 46.35) -> (-36.325, 45.85) centre (-35.825, 45.85) ccw
  arc A33 (-20.825, 45.85) -> (-21.325, 46.35) centre (-21.325, 45.85) ccw
  arc A34 (-16.775, 46.1) -> (-17.275, 45.6) centre (-16.775, 45.6) ccw
  arc A35 (-17.275, 30.1) -> (-16.775, 29.6) centre (-16.775, 30.1) ccw
  arc A36 (-2.275, 29.6) -> (-1.775, 30.1) centre (-2.275, 30.1) ccw
  arc A37 (-1.775, 45.6) -> (-2.275, 46.1) centre (-2.275, 45.6) ccw
  arc A38 (-40.375, 29.85) -> (-39.875, 30.35) centre (-40.375, 30.35) ccw
  arc A39 (-39.875, 45.85) -> (-40.375, 46.35) centre (-40.375, 45.85) ccw
  arc A40 (-54.875, 46.35) -> (-55.375, 45.85) centre (-54.875, 45.85) ccw
  arc A41 (-55.375, 30.35) -> (-54.875, 29.85) centre (-54.875, 30.35) ccw
  arc A42 (-58.925, 45.85) -> (-59.425, 46.35) centre (-59.425, 45.85) ccw
  arc A43 (-73.925, 46.35) -> (-74.425, 45.85) centre (-73.925, 45.85) ccw
  arc A44 (-74.425, 30.35) -> (-73.925, 29.85) centre (-73.925, 30.35) ccw
  arc A45 (-59.425, 29.85) -> (-58.925, 30.35) centre (-59.425, 30.35) ccw
  line L90 (-3.025, 25.9) -> (-16.025, 25.9)
  line L91 (-16.025, 25.9) -> (-16.025, 12.9)
  line L92 (-16.025, 12.9) -> (-3.025, 12.9)
  line L93 (-3.025, 12.9) -> (-3.025, 25.9)
  line L94 (-3.025, 25.9) -> (-16.025, 12.9) construction
  line L95 (-16.025, 25.9) -> (-3.025, 12.9) construction
  line L96 (-60.175, 25.9) -> (-73.175, 25.9)
  line L97 (-73.175, 25.9) -> (-73.175, 12.9)
  line L98 (-73.175, 12.9) -> (-60.175, 12.9)
  line L99 (-60.175, 12.9) -> (-60.175, 25.9)
  line L100 (-60.175, 25.9) -> (-73.175, 12.9) construction
  line L101 (-73.175, 25.9) -> (-60.175, 12.9) construction
  line L102 (-9.525, 19.4) -> (-9.525, 16.075)
  line L103 (-16.025, 22.575) -> (-3.025, 22.575)
  line L104 (-3.025, 22.575) -> (-3.025, 9.575)
  line L105 (-3.025, 9.575) -> (-16.025, 9.575)
  line L106 (-16.025, 9.575) -> (-16.025, 22.575)
  line L107 (-16.025, 22.575) -> (-3.025, 9.575) construction
  line L108 (-3.025, 22.575) -> (-16.025, 9.575) construction
  line L109 (-60.175, 22.2) -> (-73.175, 9.2) construction
  line L110 (-73.175, 22.2) -> (-60.175, 9.2) construction
  line L111 (-66.675, 19.4) -> (-66.675, 16.075)
  line L112 (-73.175, 22.575) -> (-60.175, 22.575)
  line L113 (-60.175, 22.575) -> (-60.175, 9.575)
  line L114 (-60.175, 9.575) -> (-73.175, 9.575)
  line L115 (-73.175, 9.575) -> (-73.175, 22.575)
  line L116 (-73.175, 22.575) -> (-60.175, 9.575) construction
  line L117 (-60.175, 22.575) -> (-73.175, 9.575) construction
  point P0 (-1.775, 29.6)
  point P1 (-17.275, 29.6)
  point P2 (-1.775, 46.1)
  point P3 (-20.825, 46.35)
  point P4 (-20.825, 29.85)
  point P5 (-36.325, 29.85)
  point P6 (-28.575, 38.1)
  point P7 (-39.875, 46.35)
  point P8 (-39.875, 29.85)
  point P9 (-55.375, 29.85)
  point P10 (-47.625, 38.1)
  point P11 (-58.925, 46.35)
  point P12 (-58.925, 29.85)
  point P13 (-74.425, 29.85)
  point P14 (-66.675, 38.1)
  point P15 (-9.525, 19.4)
  point P16 (-66.675, 19.4)
  point P17 (-9.525, 16.075)
  point P18 (-66.675, 16.075)
  dimension "d30" = 12
  dimension "d31" = 12
  dimension "d32" = 12
  dimension "d33" = 3.5
  dimension "d34" = 3.5
  dimension "d35" = 3.5
  dimension "d36" = 3.5
  dimension "d49" = 1.5
  dimension "d50" = 1
  dimension "d51" = 0.75
  dimension "d52" = 0.75
  dimension "d53" = 15.5
  dimension "d54" = 16.5
  dimension "d55" = 15.5
  dimension "d56" = 16.5
  dimension "d57" = 15.5
  dimension "d58" = 16.5
  dimension "d59" = 15.5
  dimension "d60" = 16.5
  dimension "d62" = 12
  dimension "d63" = 12
  dimension "d64" = 0.5
  dimension "d65" = 13
  dimension "d66" = 13
  dimension "d67" = 13
  dimension "d68" = 13
  dimension "d69" = 3.325
  dimension "d70" = 13
  dimension "d71" = 13
  dimension "d72" = 13
  dimension "d73" = 13
  dimension "d74" = 3.325
  dimension "d75" = 13
  dimension "d76" = 13
  constraint perpendicular L14 L67
  constraint perpendicular L18 L68
  constraint perpendicular L4 L69
  constraint coincident L67.end A25.centre
  constraint coincident L68.end A26.centre
  constraint coincident L69.end A27.centre
  constraint midpoint L8 L70.start
  constraint perpendicular L8 L70
  constraint midpoint L10 L71.start
  constraint perpendicular L10 L71
  constraint midpoint L9 L72.start
  constraint perpendicular L9 L72
  constraint midpoint L11 L73.start
  constraint perpendicular L11 L73
  constraint horizontal L74
  constraint vertical L75
  constraint horizontal L76
  constraint vertical L77
  constraint horizontal L78
  constraint perpendicular L78 L79
  constraint parallel L78 L80
  constraint parallel L79 L81
  constraint coincident P6 L67.start
  constraint horizontal L82
  constraint perpendicular L82 L83
  constraint parallel L82 L84
  constraint parallel L83 L85
  constraint coincident P10 L68.start
  constraint horizontal L86
  constraint perpendicular L86 L87
  constraint parallel L86 L88
  constraint parallel L87 L89
  constraint coincident P14 L69.start
  constraint coincident P4 L79
  constraint coincident P4 L80
  constraint tangent L79 A30
  constraint tangent L80 A30
  constraint coincident P5 L80
  constraint coincident P5 L81
  constraint tangent L80 A31
  constraint tangent L81 A31
  constraint equal A30 A31
  constraint tangent L78 A32
  constraint tangent L81 A32
  constraint equal A30 A32
  constraint coincident P3 L78
  constraint coincident P3 L79
  constraint tangent L78 A33
  constraint tangent L79 A33
  constraint equal A30 A33
  constraint tangent L75 A34
  constraint tangent L76 A34
  constraint equal A30 A34
  constraint coincident P1 L74
  constraint coincident P1 L75
  constraint tangent L74 A35
  constraint tangent L75 A35
  constraint equal A30 A35
  constraint coincident P0 L74
  constraint coincident P0 L77
  constraint tangent L74 A36
  constraint tangent L77 A36
  constraint equal A30 A36
  constraint coincident P2 L76
  constraint coincident P2 L77
  constraint tangent L76 A37
  constraint tangent L77 A37
  constraint equal A30 A37
  constraint coincident P8 L83
  constraint coincident P8 L84
  constraint tangent L83 A38
  constraint tangent L84 A38
  constraint equal A30 A38
  constraint coincident P7 L82
  constraint coincident P7 L83
  constraint tangent L82 A39
  constraint tangent L83 A39
  constraint equal A30 A39
  constraint tangent L82 A40
  constraint tangent L85 A40
  constraint equal A30 A40
  constraint coincident P9 L84
  constraint coincident P9 L85
  constraint tangent L84 A41
  constraint tangent L85 A41
  constraint equal A30 A41
  constraint coincident P11 L86
  constraint coincident P11 L87
  constraint tangent L86 A42
  constraint tangent L87 A42
  constraint equal A30 A42
  constraint tangent L86 A43
  constraint tangent L89 A43
  constraint equal A30 A43
  constraint coincident P13 L88
  constraint coincident P13 L89
  constraint tangent L88 A44
  constraint tangent L89 A44
  constraint equal A30 A44
  constraint coincident P12 L87
  constraint coincident P12 L88
  constraint tangent L87 A45
  constraint tangent L88 A45
  constraint equal A30 A45
  constraint horizontal L90
  constraint perpendicular L90 L91
  constraint parallel L90 L92
  constraint parallel L91 L93
  constraint coincident L94 P15
  constraint coincident L95 P15
  constraint coincident P15 A28.centre
  constraint horizontal L96
  constraint perpendicular L96 L97
  constraint parallel L96 L98
  constraint parallel L97 L99
  constraint coincident L100 P16
  constraint coincident L101 P16
  constraint coincident P16 A29.centre
  constraint vertical L102
  constraint horizontal L103
  constraint perpendicular L103 L104
  constraint parallel L103 L105
  constraint parallel L104 L106
  constraint coincident L107 P17
  constraint coincident L108 P17
  constraint coincident P17 L102.end
  constraint vertical L111
  constraint horizontal L112
  constraint perpendicular L112 L113
  constraint parallel L112 L114
  constraint parallel L113 L115
  constraint coincident L116 P18
  constraint coincident L117 P18
  constraint coincident P18 L111.end
  measures "d30" distance of P6 L67.end
  measures "d31" distance of P10 L68.end
  measures "d32" distance of P14 L69.end
  measures "d33" diameter of A24
  measures "d34" diameter of A25
  measures "d35" diameter of A26
  measures "d36" diameter of A27
  measures "d49" distance of L70.start L70.end
  measures "d50" distance of L71.start L71.end
  measures "d51" distance of L72.start L72.end
  measures "d52" distance of L73.start L73.end
  measures "d53" distance of P0 P1
  measures "d54" distance of P0 P2
  measures "d55" distance of P4 P5
  measures "d56" distance of P3 P4
  measures "d57" distance of P8 P9
  measures "d58" distance of P7 P8
  measures "d59" distance of P12 P13
  measures "d60" distance of P11 P12
  measures "d62" diameter of A28
  measures "d63" diameter of A29
  measures "d64" radius of A30
  measures "d65" distance of L91.end L92.end
  measures "d66" distance of L90.end L91.end
  measures "d67" distance of L97.end L98.end
  measures "d68" distance of L96.end L97.end
  measures "d69" distance of P15 P17
  measures "d70" distance of L104.end L105.end
  measures "d71" distance of L103.end L104.end
  measures "d72" distance of L109.end L110.end
  measures "d73" distance of L110.start L109.end
  measures "d74" distance of P16 P18
  measures "d75" distance of L113.end L114.end
  measures "d76" distance of L112.end L113.end
extrude "Extrude3" cut sketch "Sketch3" against normal blind 5 contours A6 L4 A7 L5 A8 L6 A9 L7 | A10 L8 A11 L9 A12 L10 A13 L11 | A10 L8 L11 L70 L73 L74 L77 A36 | L8 A11 L9 L70 L72 L74 L75 A35 | L10 A13 L11 L71 L73 L76 L77 A37 | L9 A12 L10 L71 L72 L75 L76 A34 | A14 L12 A15 L13 A16 L14 A17 L15 | A20 L16 A21 L17 A22 L18 A23 L19 | L78 L79 L80 L81 A30 A31 A32 A33 | L82 L83 L84 L85 A38 A39 A40 A41 | L86 L87 L88 L89 A42 A43 A44 A45 | A28 L103 | A28 L91 L92 L93 L103 L104 L106 | L92 L104 L105 L106 | A29 L112 | A29 L97 L98 L99 L112 L113 L115 | L98 L113 L114 L115 picked at (-11.3007, 20.5964) picked at (-68.567, 20.8682)
extrude "Extrude4" cut sketch "Sketch3" against normal blind 0.5 from surface at -1 contours A24 | A25 | A26 | A27
equation "d18 = 'EtchPad'"
equation "d51 = ( 1.5 / 2 ) * 1 mm"
equation "d69 = 3.7 mm - 0.375 mm"
equation "d74 = 3.7 mm - 0.375 mm"
